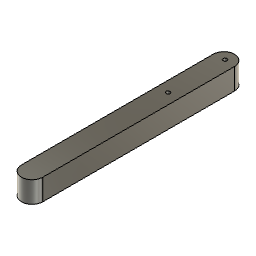
ClaspLeft v1 (Autodesk Fusion 360 design; units mm, degrees)
Autodesk Fusion 360 part; units mm, degrees
sketch "Sketch1" plane through (0, 0, 0) normal (0, 0, 1) x (1, 0, 0)
  line L0 (0, 0) -> (0, 0)
  line L1 (9.525, 9.525) -> (9.525, 180.975)
  line L2 (0, 190.5) -> (0, 190.5)
  line L3 (-9.525, 180.975) -> (-9.525, 9.525)
  line L4 (0, 0) -> (0, 190.5) construction
  arc A0 (-9.525, 9.525) -> (0, 0) centre (0, 9.525) ccw
  arc A1 (0, 0) -> (9.525, 9.525) centre (0, 9.525) ccw
  arc A2 (0, 190.5) -> (-9.525, 180.975) centre (0, 180.975) ccw
  arc A3 (9.525, 180.975) -> (0, 190.5) centre (0, 180.975) ccw
  circle A4 centre (0, 182) radius 1.75
  circle A5 centre (0, 131.2) radius 1.75
  dimension "d1" = 190.5
  dimension "d2" = 19.05
  dimension "d3" = 9.525
  dimension "d4" = 9.525
  dimension "d5" = 9.525
  dimension "d6" = 9.525
  dimension "d7" = 3.5
  dimension "d8" = 3.5
  dimension "d9" = 50.8
  constraint vertical L1
  constraint vertical L3
  constraint coincident L0.start L0.end
  constraint tangent L3 A0
  constraint tangent L1 A1
  constraint tangent L3 A2
  constraint tangent L1 A3
  constraint coincident L4 A4.centre
  constraint coincident L4 A5.centre
  measures "d1" distance of L0.start L2.start
  measures "d2" distance of L1 L3
  measures "d3" radius of A0
  measures "d4" radius of A1
  measures "d5" radius of A2
  measures "d6" radius of A3
  measures "d7" diameter of A4
  measures "d8" diameter of A5
  measures "d9" distance of A4.centre A5.centre
extrude "Extrude1" add sketch "Sketch1" along normal blind 19.05
